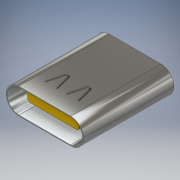
# Autodesk Inventor part: XGEN_USB-C_socket_pcb
Saved by Autodesk Inventor 2019 (Build 230136000, 136)
## iProperties
Created: 2019-03-01
Part Number: XGEN_USB-C_socket_pcb
Material: Generic
Document SubType Name: Modeling
Designer: Rene
Density: 1 g/cm^3
Appearance: Chrome - Polished
Author: Rene
Autodesk Inventor part; units mm, degrees
ref_plane "YZ Plane" through (0, 0, 0) normal (1, 0, 0) x (0, 1, 0)
ref_plane "XZ Plane" through (0, 0, 0) normal (0, 1, 0) x (-1, 0, 0)
ref_plane "XY Plane" through (0, 0, 0) normal (0, 0, 1) x (1, 0, 0)
sketch "Sketch1" plane through (0, 0, 0) normal (0, 0, 1) x (1, 0, 0)
  line L0 (-4.5, -1.5) -> (4.5, -1.5)
  line L1 (4.5, -1.5) -> (4.5, 1.5)
  line L2 (4.5, 1.5) -> (-4.5, 1.5)
  line L3 (-4.5, 1.5) -> (-4.5, -1.5)
  point P0 (0, 0)
  dimension "d0" = 3
  dimension "d1" = 1.5
  dimension "d2" = 9
  dimension "d3" = 4.5
  constraints: 8 end point, 2 parallel, 1 horizontal, 1 perpendicular
  measures "d0" distance of L2.end L0.start
  measures "d1" vertical distance of point (0, 0) L0.start
  measures "d2" distance of L0.start L0.end
  measures "d3" horizontal distance of point (0, 0) L0.start
extrude "Extrusion1" add sketch "Sketch1" along normal blind 10.5
fillet "Fillet1" radius 1.5 4 edges at (4.5, 1.5, 5.25) (4.5, -1.5, 5.25) (-4.5, -1.5, 5.25) (-4.5, 1.5, 5.25)
sketch "Sketch2" plane through (0, 0, 10.5) normal (0, 0, 1) x (1, 0, 0)
  arc A0 (-3, 1.5) -> (-3, -1.5) centre (-3, 0) ccw projected
  line L0 (-3, -1.5) -> (3, -1.5) projected
  arc A1 (3, -1.5) -> (3, 1.5) centre (3, 0) ccw projected
  line L1 (3, 1.5) -> (-3, 1.5) projected
  arc A2 (-3, 1.4) -> (-3, -1.4) centre (-3, 0) ccw
  line L2 (-3, 1.4) -> (3, 1.4)
  arc A3 (3, -1.4) -> (3, 1.4) centre (3, 0) ccw
  line L3 (3, -1.4) -> (-3, -1.4)
  point P0 (0, 0)
  dimension "d7" = 0.1
  constraints: 4 end point, 4 point on circle, 2 centre point, 3 other
  measures "d7" distance between parallel lines of L1 L2
extrude "Extrusion2" cut sketch "Sketch2" against normal blind 10 contours L2 A3 L3 A2
sketch "Sketch4" plane through (-3, 1.5, 0) normal (0, 1, 0) x (1, 0, 0)
  line L0 (2.5, -8.5) -> (2.025, -6.6503)
  line L1 (1.8313, -6.5) -> (1.6687, -6.5)
  line L2 (1.475, -6.6503) -> (1, -8.5)
  line L3 (6, -10.5) -> (0, -10.5) projected
  arc A0 (1.6687, -6.5) -> (1.475, -6.6503) centre (1.6687, -6.7) ccw
  arc A1 (2.025, -6.6503) -> (1.8313, -6.5) centre (1.8313, -6.7) ccw
  line L4 (2.3545, -8.5) -> (1.8886, -6.6853)
  arc A2 (1.8886, -6.6853) -> (1.8313, -6.6409) centre (1.8313, -6.7) ccw
  line L5 (1.8313, -6.6409) -> (1.6687, -6.6409)
  arc A3 (1.6687, -6.6409) -> (1.6114, -6.6853) centre (1.6687, -6.7) ccw
  line L6 (1.6114, -6.6853) -> (1.1455, -8.5)
  line L7 (1, -8.5) -> (1.1455, -8.5)
  line L8 (2.3545, -8.5) -> (2.5, -8.5)
  point P0 (3, 0)
  point P1 (1.9865, -6.5)
  point P2 (1.5135, -6.5)
  dimension "d11" = 0.5135
  dimension "d12" = 0.5135
  dimension "d13" = 1.5
  dimension "d14" = 2
  dimension "d15" = 2
  dimension "d16" = 1
  dimension "d17" = 0.4729
  dimension "d18" = 0.2
  constraints: 16 end point, 8 point on circle, 4 centre point, 4 point on line, 4 tangent, 3 horizontal, 1 equal radius, 2 other
  measures "d11" horizontal distance of point (1.986, -6.5) L0.start
  measures "d12" horizontal distance of point (1.514, -6.5) L2.end
  measures "d13" distance of L2.end L0.start
  measures "d14" distance from line of L2.end L3
  measures "d15" vertical distance of point (1.514, -6.5) L2.end
  measures "d16" horizontal distance of L3.end L2.end
  measures "d17" distance of point (1.986, -6.5) point (1.514, -6.5)
  measures "d18" radius of A0
extrude "Extrusion3" cut sketch "Sketch4" against normal blind 1
mirror "Mirror2" about plane through (0, 0, 0) normal (1, 0, 0) of "Extrusion3"
sketch "Sketch5" plane through (0, 0, 0.5) normal (0, 0, 1) x (1, 0, 0)
  arc A0 (-3, 1.4) -> (-3, -1.4) centre (-3, 0) ccw projected
  line L0 (3, -1.4) -> (-3, -1.4) projected
  arc A1 (3, -1.4) -> (3, 1.4) centre (3, 0) ccw projected
  line L1 (-3, 1.4) -> (3, 1.4) projected
  arc A2 (-3, 1.35) -> (-3, -1.35) centre (-3, 0) ccw
  line L2 (-3, 1.35) -> (3, 1.35)
  arc A3 (3, -1.35) -> (3, 1.35) centre (3, 0) ccw
  line L3 (3, -1.35) -> (-3, -1.35)
  point P0 (0, 0)
  dimension "d21" = 0.05
  constraints: 4 end point, 4 point on circle, 2 centre point, 3 other
  measures "d21" distance between parallel lines of L1 L2
extrude "Extrusion4" add sketch "Sketch5" along normal blind 4 contours L2 A3 L3 A2
sketch "Sketch6" plane through (0, 0, 4.5) normal (0, 0, 1) x (1, 0, 0)
  line L0 (-3, 0.5) -> (3, 0.5)
  line L1 (3, 0.5) -> (3, -0.5)
  line L2 (3, -0.5) -> (-3, -0.5)
  line L3 (-3, -0.5) -> (-3, 0.5)
  point P0 (0, 0)
  dimension "d24" = 1
  dimension "d25" = 0.5
  dimension "d26" = 6
  dimension "d27" = 3
  constraints: 8 end point, 2 parallel, 1 horizontal, 1 perpendicular
  measures "d24" distance of L2.end L0.start
  measures "d25" vertical distance of point (0, 0) L2.end
  measures "d26" distance of L1.end L2.end
  measures "d27" horizontal distance of point (0, 0) L2.end
extrude "Extrusion5" add sketch "Sketch6" along normal blind 5
fillet "Fillet2" radius 0.3 4 edges at (-3, 0.5, 7) (-3, -0.5, 7) (3, 0.5, 7) (3, -0.5, 7)
equation "\"d1\" = 0.5 * d0"
equation "\"d3\" = 0.5 * d2"
equation "\"d12\" = d11"
equation "\"d25\" = 0.5 * d24"
equation "\"d27\" = 0.5 * d26"
body "Solid1"
